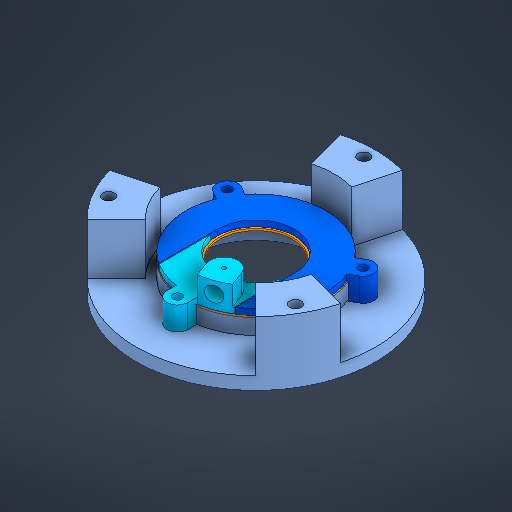
# Autodesk Inventor part: WellyBottle-Adapter
Saved by Autodesk Inventor 2026 (Build 300175050, 175E)
## iProperties
Created: 2024-06-05
Part Number: WellyBottle-Adapter
Material: Generic
Document SubType Name: Modeling
Designer: incep
Density: 1 g/cm^3
Appearance: Default
Author: incep
## iProperties of the stored document WellyBottle-Adapter_3DPrint.ipt
Created: 2024-06-05
Part Number: WellyBottle-Adapter_3DPrint
Material: Generic
Document SubType Name: Modeling
Designer: incep
Density: 1 g/cm^3
Appearance: Default
Author: incep
Autodesk Inventor part; units mm, degrees
ref_plane "YZ Plane" through (0, 0, 0) normal (1, 0, 0) x (0, 1, 0)
ref_plane "XZ Plane" through (0, 0, 0) normal (0, 1, 0) x (-1, 0, 0)
sketch "Sketch1" plane through (0, 0, 0) normal (0, 1, 0) x (-1, 0, 0)
  circle A0 centre (0, 0) radius 32 construction
  circle A1 centre (0, 0) radius 32.75
  circle A2 centre (0, 0) radius 60.865
  dimension "d0" = 64
  dimension "d1" = 0.75
  dimension "d2" = 121.73
  constraints: 3 centre point, 2 coincident
  measures "d0" diameter of A0
  measures "d1" radial gap between concentric circles of A0 A1
  measures "d2" diameter of A2
extrude "Extrusion1" add sketch "Sketch1" along normal blind 6.5
sketch "Sketch2" plane through (0, 6.5, 0) normal (0, 1, 0) x (1, 0, 0)
  circle A0 centre (0, 0) radius 55 construction
  line L0 (0, 0) -> (0, 55) construction
  circle A1 centre (0, 55) radius 2.9
  line L1 (0, 0) -> (15.753021, 58.791075)
  circle A2 centre (0, 0) radius 60.865
  line L2 (0, 0) -> (-15.753021, 58.791075)
  circle A3 centre (0, 0) radius 32.75
  circle A4 centre (0, 0) radius 60.865
  circle A5 centre (0, 0) radius 39.85
  point P0 (-8.476324, 31.634071)
  point P1 (8.476324, 31.634071)
  point P2 (-10.313939, 38.492144)
  point P3 (10.313939, 38.492144)
  dimension "d5" = 110
  dimension "d6" = 5.8
  dimension "d7" = 15
  dimension "d11" = 79.7
  constraints: 6 end point, 3 coincident, 2 centre point, 1 symmetric about line, 1 vertical, 1 vertical alignment, 4 other
  measures "d6" diameter of A1
  measures "d7" angle of L0 L1
  measures "d11" diameter of A5
extrude "Extrusion2" add sketch "Sketch2" along normal blind 26.1 contours A5 L2 A2 L1 picked at (-9.544927, 50.311841)
pattern_circular "Circular Pattern1" count 3 over 360 about axis through (0, -10, 0) along (0, 1, 0) of "Extrusion2"
sketch "Sketch3" plane through (0, 6.5, 0) normal (0, 1, 0) x (1, 0, 0)
  circle A0 centre (0, 0) radius 32.75 projected
  circle A1 centre (0, 0) radius 35.75
  dimension "d15" = 3
  constraints: 1 centre point
  measures "d15" radial gap between concentric circles of A0 A1
extrude "Extrusion3" add sketch "Sketch3" along normal blind 8.9
sketch "Sketch4" plane through (0, 6.5, 0) normal (0, 1, 0) x (1, 0, 0)
  circle A0 centre (0, 0) radius 40 construction
  circle A1 centre (0, -40) radius 2.9
  dimension "d18" = 80
  dimension "d19" = 5.8
  constraints: 1 centre point, 1 coincident, 1 vertical alignment, 2 other
  measures "d19" diameter of A1
extrude "Extrusion4" cut sketch "Sketch4" against normal up to surface (6.5 mm away)
pattern_circular "Circular Pattern2" count 3 over 360 about axis through (0, -10, 0) along (0, 1, 0) of "Extrusion4"
sketch "Sketch5" plane through (0, 15.4, 0) normal (0, 1, 0) x (1, 0, 0)
  circle A0 centre (0, 0) radius 35.75
  circle A1 centre (-47.631397, -27.5) radius 2.9
  circle A2 centre (47.631397, -27.5) radius 2.9
  circle A3 centre (0, 0) radius 19.05 construction
  circle A4 centre (0, 0) radius 19.55
  line L0 (-19.55, 0) -> (-19.55, -29.93092)
  circle A5 centre (0, 0) radius 35.75 construction
  line L1 (19.55, 0) -> (19.55, -29.93092)
  circle A6 centre (-34.641016, 20) radius 2.9 construction
  circle A7 centre (-34.641016, 20) radius 2.3
  arc A8 (-31.991016, 24.589935) -> (-37.291016, 15.410065) centre (-34.641016, 20) ccw
  line L2 (-37.291016, 15.410065) -> (-33.268285, 13.08754)
  line L3 (-31.991016, 24.589935) -> (-27.968285, 22.26741)
  circle A9 centre (0, 0) radius 36.25
  line L4 (-19.05, -4.393177) -> (-19.05, -30.251612)
  line L5 (19.05, -4.393177) -> (19.05, -30.251612)
  circle A10 centre (0, -40) radius 2.9
  circle A11 centre (0, -40) radius 2.3
  line L6 (5.3, -40) -> (5.3, -35.35495)
  line L7 (-5.3, -40) -> (-5.3, -35.35495)
  arc A12 (-5.3, -40) -> (5.3, -40) centre (0, -40) ccw
  point P0 (-33.706068, 13.340295)
  point P1 (-28.406068, 22.520164)
  point P2 (5.3, -35.860459)
  point P3 (-5.3, -35.860459)
  dimension "d25" = 38.1
  dimension "d26" = 0.5
  dimension "d27" = 4.6
  dimension "d28" = 3
  dimension "d39" = 0.5
  dimension "d47" = 0.5
  dimension "d48" = 0.5
  dimension "d49" = 4.6
  constraints: 16 end point, 8 point on circle, 7 centre point, 6 parallel, 5 coincident, 5 tangent, 3 vertical, 9 other
  measures "d25" diameter of A3
  measures "d26" radial gap between concentric circles of A3 A4
  measures "d27" diameter of A7
  measures "d28" radial gap between concentric circles of A8 A7
  measures "d39" radial gap between concentric circles of A0 A9
  measures "d47" distance between parallel lines of L0 L4
  measures "d48" distance between parallel lines of L1 L5
  measures "d49" diameter of A11
sketch "Sketch5 outline for Extrusion5" plane through (0, 15.4, 0) normal (0, 1, 0) x (1, 0, 0)
  line L0 (19.55, 0) -> (19.55, -29.93092)
  arc A0 (-19.55, 0) -> (19.55, 0) centre (0, 0) cw
  line L1 (-19.55, -29.93092) -> (-19.55, 0)
  arc A1 (19.55, -29.93092) -> (-19.55, -29.93092) centre (0, 0) ccw
extrude "Extrusion5" add sketch "Sketch5 outline for Extrusion5" along normal blind 3 separate body
extrude "Extrusion8" add sketch "Sketch5" along normal blind 3 contours A0 L2 A9 L3 | A9 L2 A8 L3 bodies 2
extrude "Extrusion9" add sketch "Sketch5" against normal up to surface (8.9 mm away) contours A9 L2 A8 L3 bodies 2
pattern_circular "Circular Pattern4" count 2 over 120 about axis through (0, -10, 0) along (0, -1, 0) of "Extrusion9", "Extrusion8" bodies 2
extrude "Extrusion10" add sketch "Sketch5" along normal blind 3 separate body contours A0 L4 A4 L5 | L6 A9 L7 A0 | A9 L6 A12 L7 | A10
extrude "Extrusion11" add sketch "Sketch5" against normal up to surface (8.9 mm away) contours A9 L6 A12 L7 | A10 bodies 3
sketch "Sketch7" plane through (0, 18.4, 0) normal (0, 1, 0) x (1, 0, 0)
  point P0 (0, 0)
sketch "Sketch8" plane through (0, 15.4, 0) normal (0, -1, 0) x (1, 0, 0)
  circle A0 centre (0, 0) radius 32.75 construction
  circle A1 centre (0, 0) radius 27.3 construction
  circle A2 centre (9.33715, 25.653609) radius 1
  line L0 (0, 0) -> (9.33715, 25.653609) construction
  line L1 (0, 0) -> (0, 27.3) construction
  dimension "d55" = 5.45
  dimension "d56" = 2
  dimension "d57" = 20
  constraints: 4 end point, 2 centre point, 2 point on circle, 1 vertical
  measures "d55" radial gap between concentric circles of A0 A1
  measures "d56" diameter of A2
  measures "d57" angle of L1 L0
extrude "Extrusion12" cut sketch "Sketch8" against normal up to surface (3 mm away) bodies 3
sketch "Sketch9" plane through (0, 18.4, 0) normal (0, 1, 0) x (1, 0, 0)
  circle A0 centre (9.33715, -25.653609) radius 1
  circle A1 centre (9.33715, -25.653609) radius 1 construction
  arc A2 (15.914998, -23.259468) -> (2.759302, -28.04775) centre (9.33715, -25.653609) ccw
  line L0 (9.33715, -25.653609) -> (12.22722, -33.594011) construction
  circle A3 centre (0, 0) radius 35.75 construction
  line L1 (15.914998, -23.259468) -> (18.568386, -30.549591)
  line L2 (2.759302, -28.04775) -> (5.41269, -35.337873)
  arc A4 (5.3, -35.35495) -> (19.05, -30.251612) centre (0, 0) ccw
  dimension "d60" = 6
  constraints: 6 end point, 6 point on circle, 2 line through centre, 2 parallel, 2 tangent, 1 centre point, 1 coincident, 1 point on line
  measures "d60" radial gap between concentric circles of A2 A0
extrude "Extrusion13" add sketch "Sketch9" along normal blind 10 bodies 3
ref_plane "Work Plane1" through (12.22722, 28.4, 33.594011) normal (0.3420201, 0, 0.9396926) x (0, 1, 0)
sketch "Sketch10" plane through (12.22722, 28.4, 33.594011) normal (0.3420201, 0, 0.9396926) x (0, 1, 0)
  circle A0 centre (-6, 0) radius 3.85
  circle A1 centre (-6, 0) radius 1.5
  line L0 (0, -7) -> (0, 7) projected
  point P0 (-28.4, 0)
  dimension "d63" = 7.7
  dimension "d66" = 3
  dimension "d67" = 6
  constraints: 2 centre point, 1 coincident
  measures "d63" diameter of A0
  measures "d66" diameter of A1
  measures "d67" distance from line of L0 A0.centre
extrude "Extrusion14" cut sketch "Sketch10" against normal blind 11 contours A0 | A1 bodies 3
extrude "Extrusion15" cut sketch "Sketch10" against normal blind 20 contours A1 bodies 3
sketch "Sketch11" plane through (0, 15.4, 0) normal (0, -1, 0) x (1, 0, 0)
  arc A0 (19.05, 30.251612) -> (5.3, 35.35495) centre (0, 0) ccw
  arc A1 (19.05, 4.393177) -> (-19.05, 4.393177) centre (0, 0) ccw
  circle A2 centre (0, 0) radius 18.55
  circle A3 centre (9.33715, 25.653609) radius 1
  circle A4 centre (0, 0) radius 35.75
  point P0 (5.3, 35.35495)
  dimension "d70" = 1
  constraints: 2 centre point, 2 coincident, 1 concentric
  measures "d70" radial gap between concentric circles of A1 A2
extrude "Extrusion16" add sketch "Sketch11" along normal blind 1 separate body
